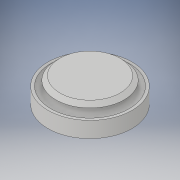
# Autodesk Inventor part: Diaphragme2
Saved by Autodesk Inventor 2018 (Build 220112000, 112)
## iProperties
Created: 2020-03-27
Part Number: Diaphragme2
Material: Generic
Document SubType Name: Modeling
Designer: emile
Density: 1 g/cm^3
Appearance: Default
Author: emile
Autodesk Inventor part; units mm, degrees
ref_plane "YZ Plane" through (0, 0, 0) normal (1, 0, 0) x (0, 1, 0)
ref_plane "XZ Plane" through (0, 0, 0) normal (0, 1, 0) x (-1, 0, 0)
ref_plane "XY Plane" through (0, 0, 0) normal (0, 0, 1) x (1, 0, 0)
sketch "Sketch1" plane through (0, 0, 0) normal (0, 0, 1) x (1, 0, 0)
  line L0 (0, 0) -> (0, 6.35)
  line L1 (16.8697, 0) -> (0, 0)
  circle A0 centre (14.2875, 6.9428) radius 1.5875
  line L2 (0, 6.35) -> (12.8148, 6.35)
  line L3 (16.8697, 0) -> (16.8697, 6.35)
  line L4 (16.8697, 6.35) -> (15.7602, 6.35)
  line L5 (13.6947, 8.4155) -> (0, 8.4155)
  line L6 (0, 8.4155) -> (0, 6.35)
  line L7 (13.6947, 8.4155) -> (15.7602, 6.35) construction
  line L8 (13.6947, 8.4155) -> (13.6947, 10.003)
  line L9 (13.6947, 10.003) -> (0, 10.003)
  line L10 (0, 10.003) -> (0, 8.4155)
  dimension "d0" = 3.175
  dimension "d5" = 45
  dimension "d6" = 1.5875
  dimension "d7" = 3.175
  dimension "d8" = 6.35
  dimension "d13" = 14.2875
  dimension "d14" = 2.921
  constraints: 22 end point, 5 perpendicular, 3 point on circle, 3 vertical, 2 horizontal, 1 centre point, 1 horizontal alignment
  measures "d0" diameter of A0
  measures "d5" angle of L4 L7
  measures "d6" distance of L5.start L8.end
  measures "d7" distance between parallel lines of L8 L3
  measures "d8" distance of L1.start L3.end
  measures "d13" distance from line of L0 A0.centre
  measures "d14" distance of L5.start L4.end
revolve "Revolution1" add sketch "Sketch1" angle 360 about axis through (0, 10.003, 0) along (0, -1, 0) contours L0 L2 A0 L4 L3 L1 | L6 L5 A0 L2 | L10 L9 L8 L5
chamfer "Chamfer1" distance 1.5875 angle 45 1 edges at (-13.6947, 10.003, 0)
sketch "Sketch2" plane through (0, 10.003, 0) normal (0, 1, 0) x (1, 0, 0)
  circle A0 centre (0, 0) radius 12.1072 projected
  point P0 (0, 0)
sketch "Sketch4" plane through (0, 10.003, 0) normal (0, 1, 0) x (1, 0, 0)
  circle A0 centre (0, 0) radius 3.1115
  circle A1 centre (0, 7.62) radius 1.905
  circle A2 centre (-6.5991, 3.81) radius 1.905
  circle A3 centre (-6.5991, -3.81) radius 1.905
  circle A4 centre (0, -7.62) radius 1.905
  circle A5 centre (6.5991, -3.81) radius 1.905
  circle A6 centre (6.5991, 3.81) radius 1.905
  dimension "d17" = 6.223
  dimension "d18" = 7.62
  dimension "d19" = 3.81
  dimension "d22" = 360
  constraints: 7 centre point, 1 coincident, 1 vertical alignment, 13 other
  measures "d17" diameter of A0
  measures "d18" distance of A0.centre A1.centre
  measures "d19" diameter of A1
body "Solid1"
